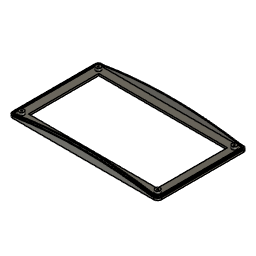
Case -  v1 v3 (Autodesk Fusion 360 design; units mm, degrees)
Autodesk Fusion 360 part; units mm, degrees
sketch "sketch_ecran_base" plane through (0, 0, 0) normal (0, 0, 1) x (1, 0, 0)
  line L0 (5, 0) -> (186, 0)
  line L1 (191, 5) -> (191, 110)
  line L2 (186, 115) -> (5, 115)
  line L3 (0, 110) -> (0, 5)
  arc A0 (5, 115) -> (0, 110) centre (5, 110) ccw
  arc A1 (191, 110) -> (186, 115) centre (186, 110) ccw
  arc A2 (186, 0) -> (191, 5) centre (186, 5) ccw
  arc A3 (0, 5) -> (5, 0) centre (5, 5) ccw
  line L4 (6.5, 111.5) -> (184.5, 111.5)
  line L5 (187, 109) -> (187, 6)
  line L6 (184.5, 3.5) -> (6.5, 3.5)
  line L7 (4, 6) -> (4, 109)
  arc A4 (6.5, 111.5) -> (4, 109) centre (6.5, 109) ccw
  arc A5 (187, 109) -> (184.5, 111.5) centre (184.5, 109) ccw
  arc A6 (184.5, 3.5) -> (187, 6) centre (184.5, 6) ccw
  arc A7 (4, 6) -> (6.5, 3.5) centre (6.5, 6) ccw
  point P0 (191, 0)
  point P1 (0, 115)
  point P2 (4, 111.5)
  point P3 (187, 111.5)
  point P4 (4, 3.5)
  dimension "d1" = 191
  dimension "d2" = 115
  dimension "d3" = 5
  dimension "d4" = 5
  dimension "d5" = 183
  dimension "d6" = 108
  dimension "d7" = 2.5
  dimension "d8" = 2.5
  dimension "d9" = 4
  dimension "d10" = 3.5
  constraint horizontal L0
  constraint vertical L1
  constraint horizontal L2
  constraint vertical L3
  constraint coincident P1 L2
  constraint coincident P1 L3
  constraint tangent L2 A0
  constraint tangent L3 A0
  constraint tangent L2 A1
  constraint tangent L1 A1
  constraint coincident P0 L1
  constraint coincident P0 L0
  constraint tangent L1 A2
  constraint tangent L0 A2
  constraint equal A1 A2
  constraint coincident origin L3
  constraint coincident origin L0
  constraint tangent L3 A3
  constraint tangent L0 A3
  constraint equal A1 A3
  constraint horizontal L4
  constraint vertical L5
  constraint horizontal L6
  constraint vertical L7
  constraint coincident P2 L4
  constraint coincident P2 L7
  constraint tangent L4 A4
  constraint tangent L7 A4
  constraint coincident P3 L4
  constraint coincident P3 L5
  constraint tangent L4 A5
  constraint tangent L5 A5
  constraint tangent L6 A6
  constraint tangent L5 A6
  constraint equal A5 A6
  constraint coincident P4 L6
  constraint coincident P4 L7
  constraint tangent L6 A7
  constraint tangent L7 A7
  constraint equal A5 A7
  measures "d1" distance of origin P0
  measures "d2" distance of origin P1
  measures "d3" radius of A0
  measures "d4" radius of A1
  measures "d5" distance of P2 P3
  measures "d6" distance of P2 P4
  measures "d7" radius of A4
  measures "d8" radius of A5
  measures "d9" distance of L3 L7
  measures "d10" distance of L2 L4
extrude "Extrude1" add sketch "sketch_ecran_base" along normal blind 15 contours L0 L1 L2 L3 A0 A1 A2 A3 | L4 L5 L6 L7 A4 A5 A6 A7 makes body 1
extrude "Extrude2" add sketch "sketch_ecran_base" along normal blind 0.4 from surface at 15 contours L4 L5 L6 L7 A4 A5 A6 A7 bodies 1
sketch "sketch_ecran_sides" plane through (0, 0, 0) normal (0, -1, 0) x (1, 0, 0)
  line L0 (5, 0) -> (186, 0)
  line L1 (186, 0) -> (186, 15)
  line L2 (186, 15) -> (5, 15)
  line L3 (5, 15) -> (5, 0)
  line L4 (95.5, 15) -> (95.5, 7) construction
  arc A0 (186, 0) -> (5, 0) centre (95.5, -581.5179) ccw
  dimension "d16" = 8
  constraint midpoint L2 L4.start
  constraint perpendicular L2 L4
  constraint coincident L4.end A0
  constraint coincident L0.end L1.start
  constraint coincident L0.start L3.end
  measures "d16" distance of L4.start L4.end
extrude "Extrude3" cut sketch "sketch_ecran_sides" against normal blind 125 contours L0 A0 bodies 1
chamfer "Chamfer1" distance 1.3 distance2 1.8 8 edges at (0, 57.5, 15) (1.4645, 1.4645, 15) (95.5, 0, 15) (189.5355, 1.4645, 15) (191, 57.5, 15) (189.5355, 113.5355, 15) (95.5, 115, 15) (1.4645, 113.5355, 15) measured on face at (189.6667, 74.6667, 15) measured on face at (189.6667, 74.6667, 15) measured on face at (189.6667, 74.6667, 15) measured on face at (189.6667, 74.6667, 15) measured on face at (189.6667, 74.6667, 15) measured on face at (189.6667, 74.6667, 15) measured on face at (189.6667, 74.6667, 15) measured on face at (189.6667, 74.6667, 15) on bodies 1
sketch "sketch_backplate_base" plane through (0, 0, 0) normal (0, 0, 1) x (1, 0, 0)
  line L0 (5, 0) -> (186, 0)
  line L1 (191, 5) -> (191, 110)
  line L2 (186, 115) -> (5, 115)
  line L3 (0, 110) -> (0, 5)
  circle A0 centre (8.25, 106.75) radius 3.25
  circle A1 centre (8.25, 106.75) radius 2
  circle A2 centre (8.25, 106.75) radius 1
  line L4 (95.5, 115) -> (95.5, 0) construction
  line L5 (0, 57.5) -> (191, 57.5) construction
  circle A3 centre (182.75, 106.75) radius 3.25
  circle A4 centre (182.75, 106.75) radius 2
  circle A5 centre (182.75, 106.75) radius 1
  circle A6 centre (8.25, 8.25) radius 3.25
  circle A7 centre (8.25, 8.25) radius 2
  circle A8 centre (8.25, 8.25) radius 1
  circle A9 centre (182.75, 8.25) radius 3.25
  circle A10 centre (182.75, 8.25) radius 2
  circle A11 centre (182.75, 8.25) radius 1
  arc A12 (5, 115) -> (0, 110) centre (5, 110) ccw
  arc A13 (191, 110) -> (186, 115) centre (186, 110) ccw
  arc A14 (186, 0) -> (191, 5) centre (186, 5) ccw
  arc A15 (0, 5) -> (5, 0) centre (5, 5) ccw
  line L6 (1.4, 110) -> (1.4, 5)
  arc A16 (1.4, 5) -> (5, 1.4) centre (5, 5) ccw
  line L7 (5, 1.4) -> (186, 1.4)
  arc A17 (186, 1.4) -> (189.6, 5) centre (186, 5) ccw
  line L8 (189.6, 5) -> (189.6, 110)
  arc A18 (189.6, 110) -> (186, 113.6) centre (186, 110) ccw
  line L9 (186, 113.6) -> (5, 113.6)
  arc A19 (5, 113.6) -> (1.4, 110) centre (5, 110) ccw
  line L10 (5, 2.8) -> (186, 2.8)
  arc A20 (186, 2.8) -> (188.2, 5) centre (186, 5) ccw
  line L11 (188.2, 5) -> (188.2, 110)
  arc A21 (188.2, 110) -> (186, 112.2) centre (186, 110) ccw
  line L12 (186, 112.2) -> (5, 112.2)
  arc A22 (5, 112.2) -> (2.8, 110) centre (5, 110) ccw
  line L13 (2.8, 110) -> (2.8, 5)
  arc A23 (2.8, 5) -> (5, 2.8) centre (5, 5) ccw
  line L14 (13, 102.5) -> (178, 102.5)
  line L15 (178, 102.5) -> (178, 12.5)
  line L16 (178, 12.5) -> (13, 12.5)
  line L17 (13, 12.5) -> (13, 102.5)
  point P0 (191, 0)
  point P1 (0, 115)
  point P2 (13, 57.5)
  point P3 (178, 57.5)
  point P4 (95.5, 102.5)
  dimension "d21" = 191
  dimension "d22" = 115
  dimension "d23" = 6.5
  dimension "d24" = 8.25
  dimension "d25" = 8.25
  dimension "d26" = 4
  dimension "d27" = 2
  dimension "d28" = 5
  dimension "d29" = -1.4
  dimension "d30" = -2.8
  dimension "d57" = 165
  dimension "d58" = 90
  constraint horizontal L0
  constraint vertical L1
  constraint horizontal L2
  constraint vertical L3
  constraint concentric A0 A1
  constraint concentric A1 A2
  constraint symmetric A0 L4 A3
  constraint symmetric A1 L4 A4
  constraint symmetric A2 L4 A5
  constraint symmetric A0 L5 A6
  constraint symmetric A1 L5 A7
  constraint symmetric A2 L5 A8
  constraint symmetric L5 A3 A9
  constraint symmetric L5 A4 A10
  constraint symmetric L5 A5 A11
  constraint coincident L2 L4.start
  constraint coincident L3 L5.start
  constraint coincident P1 L2
  constraint coincident P1 L3
  constraint tangent L2 A12
  constraint tangent L3 A12
  constraint coincident L1 L5.end
  constraint tangent L1 A13
  constraint tangent L2 A13
  constraint equal A12 A13
  constraint coincident L0 L4.end
  constraint coincident P0 L0
  constraint coincident P0 L1
  constraint tangent L0 A14
  constraint tangent L1 A14
  constraint equal A12 A14
  constraint coincident origin L0
  constraint coincident origin L3
  constraint tangent L0 A15
  constraint tangent L3 A15
  constraint equal A12 A15
  constraint midpoint L3 L5.start
  constraint midpoint L1 L5.end
  constraint midpoint L2 L4.start
  constraint midpoint L0 L4.end
  constraint horizontal L14
  constraint vertical L15
  constraint horizontal L16
  constraint vertical L17
  constraint coincident L17 P2
  constraint midpoint L17 P2
  constraint coincident L15 P3
  constraint midpoint L15 P3
  constraint coincident L5 P3
  constraint coincident L14 P4
  constraint midpoint L14 P4
  constraint coincident L4 P4
  measures "d21" distance of origin P0
  measures "d22" distance of origin P1
  measures "d23" diameter of A0
  measures "d24" distance of L2 A0.centre
  measures "d25" distance of L3 A0.centre
  measures "d26" diameter of A1
  measures "d27" diameter of A2
  measures "d28" radius of A12
  measures "d57" distance of L14.start L14.end
  measures "d58" distance of L14.end L15.end
sketch "sketch_backplate_side" plane through (0, 0, 0) normal (0, 1, 0) x (1, 0, 0)
  line L0 (0, 0) -> (191, 0)
  line L1 (95.5, 0) -> (95.5, -11.2) construction
  line L2 (0, 0) -> (0, -2.4)
  line L3 (0, -2.4) -> (8.25, -2.4)
  line L4 (8.25, 0) -> (8.25, -2.4)
  line L5 (0, -2.4) -> (0, -3.9)
  line L6 (0, -3.9) -> (8.25, -3.9)
  line L7 (8.25, -2.4) -> (8.25, -3.9)
  line L8 (191, -3.9) -> (182.75, -3.9)
  line L9 (191, -2.4) -> (182.75, -2.4)
  line L10 (191, 0) -> (191, -2.4)
  line L11 (191, -2.4) -> (191, -3.9)
  arc A0 (8.25, -2.4) -> (182.75, -2.4) centre (95.5, 562.3517) ccw
  arc A1 (8.25, -3.9) -> (182.75, -3.9) centre (95.5, 513.8584) ccw
  line L12 (182.75, 0) -> (182.75, -2.4)
  line L13 (182.75, -2.4) -> (182.75, -3.9)
  point P0 (8.25, 0)
  point P1 (182.75, 0)
  point P2 (95.5, -9.1)
  dimension "d31" = 191
  dimension "d32" = 8.25
  dimension "d33" = 11.2
  dimension "d34" = 2.4
  dimension "d35" = 1.5
  dimension "d36" = 9.1
  constraint coincident L0.start L2.start
  constraint horizontal L0
  constraint coincident L0 P0
  constraint midpoint L0 L1.start
  constraint perpendicular L0 L1
  constraint symmetric P0 L1 P1
  constraint perpendicular L0 L2
  constraint perpendicular L2 L3
  constraint coincident P0 L4.start
  constraint coincident L3 L4.end
  constraint perpendicular L3 L4
  constraint perpendicular L3 L5
  constraint perpendicular L5 L6
  constraint coincident L6 L7.end
  constraint vertical L7
  constraint symmetric L1 L0.start L0.end
  constraint symmetric L1 L2.end L9.start
  constraint symmetric L1 L3.end L9.end
  constraint symmetric L1 L5.end L8.start
  constraint symmetric L1 L6.end L8.end
  constraint coincident L1 P2
  constraint coincident P2 A0
  constraint coincident L1.end A1
  constraint symmetric L1 P0 P1
  measures "d31" distance of L0.start L0.end
  measures "d32" distance of L0.start L4.start
  measures "d33" distance of L1.start L1.end
  measures "d34" distance of L0.start L2.end
  measures "d35" distance of L2.end L5.end
  measures "d36" distance of L1.start P2
extrude "Extrude4" add sketch "sketch_backplate_base" along normal blind 3.9 separate body contours L6 A16 L7 A17 L8 A18 L9 A19 makes body 2
extrude "Extrude5" add sketch "sketch_backplate_base" along normal blind 2.4 contours L0 L1 L2 L3 A12 A13 A14 A15 | L10 A20 L11 A21 L12 A22 L13 A23 bodies 2
extrude "Extrude6" add sketch "sketch_backplate_side" along normal blind 2.8 contours L0 L4 A0 L12 bodies 2
extrude "Extrude7" add sketch "sketch_backplate_side" against normal blind 1.4 from surface at 2.8 contours L7 A0 A1 L13 bodies 2
extrude "Extrude8" add sketch "sketch_backplate_side" against normal blind 2.8 from surface at 115 contours L0 L4 A0 L12 | L7 A0 A1 L13 bodies 2
extrude "Extrude9" cut sketch "sketch_backplate_side" against normal blind 1.4 from surface at 115 contours L7 A0 A1 L13 bodies 2
extrude "Extrude10" add sketch "sketch_backplate_base" along normal blind 5.8 contours A0 | A3 | A6 | A9 bodies 2
extrude "Extrude11" add sketch "sketch_backplate_base" against normal blind 1.2 from surface at 5.8 contours A1 | A4 | A7 | A10 bodies 2
hidden bodies 1
equation "d9 = ( ( 191 - 183 ) / 2 ) * 1 mm"
equation "d10 = ( ( 115 - 108 ) / 2 ) * 1 mm"
equation "d24 = 5 mm + ( ( 6.5 / 2 ) * 1 mm )"
equation "d25 = 5 mm + ( ( 6.5 / 2 ) * 1 mm )"
equation "d32 = 5 mm + ( ( 6.5 / 2 ) * 1 mm )"
named bodies: "body_ecran", "body_backplate"
